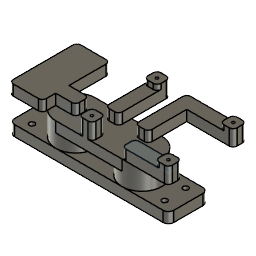
Halterung_Raspberry_Pi_5_XL4015 (Autodesk Fusion 360 design; units mm, degrees)
part number: 2026-02-12-18-16-56-274
Autodesk Fusion 360 part; units mm, degrees
note: some values were not read from the file. Set by a fixed rule: which sketch regions a step uses.
sketch "Skizze1" plane through (0, 0, 0) normal (0, 0, 1) x (1, 0, 0)
  line L0 (-35, 20) -> (85, 20)
  line L1 (85, 20) -> (85, -10)
  line L2 (85, -10) -> (-35, -10)
  line L3 (-35, -10) -> (-35, 20)
  dimension "d1" = 120
  dimension "d2" = 30
  constraint horizontal L0
  constraint vertical L1
  constraint horizontal L2
  constraint vertical L3
  measures "d1" distance of L0.start L0.end
  measures "d2" distance of L0.start L2.end
extrude "Extrusion1" add sketch "Skizze1" along normal blind 8
sketch "Skizze2" plane through (0, 0, 8) normal (0, 0, 1) x (-1, 0, 0)
  line L0 (35, 10) -> (-85, 10)
  line L1 (-85, 10) -> (-85, -20)
  line L2 (-85, -20) -> (35, -20)
  line L3 (35, -20) -> (35, 10)
  point P0 (25, -12.9992)
  point P1 (24.845, 3)
  point P2 (-75, -12.9991)
  point P3 (-75.16, 3.0001)
  dimension "d5" = 100
  dimension "d6" = 16
  dimension "d7" = 16
  dimension "d8" = 10
  dimension "d9" = 10
  dimension "d10" = 7
  measures "d5" distance of P0 P2
  measures "d6" distance of P2 P3
  measures "d7" distance of P0 P1
  measures "d8" distance of L3 P0
  measures "d9" distance of L1 P2
  measures "d10" distance of L0 P1
hole "Bohrung1" at (-25, 12.9992, 8) at (-24.845, -3, 8) at (75, 12.9991, 8) at (75.16, -3.0001, 8) direction (0, 0, -1) diameter 4 depth 45 tip angle 118
sketch "Skizze3" plane through (0, 0, 8) normal (0, 0, 1) x (-1, 0, 0)
  circle A0 centre (-75, -12.9991) radius 2
  circle A1 centre (25, -12.9992) radius 2
  circle A2 centre (24.845, 3) radius 2
  circle A3 centre (-75.16, 3.0001) radius 2
  line L0 (35, 10) -> (-85, 10)
  line L1 (-85, 10) -> (-85, -20)
  line L2 (-85, -20) -> (35, -20)
  line L3 (35, -20) -> (35, 10)
  circle A4 centre (0, -5) radius 15
  circle A5 centre (-50, -5) radius 15
  dimension "d14" = 30
  dimension "d15" = 30
  dimension "d16" = 35
  dimension "d17" = 35
  measures "d14" diameter of A4
  measures "d15" diameter of A5
  measures "d16" distance of L3 A4.centre
  measures "d17" distance of L1 A5.centre
extrude "Extrusion2" add sketch "Skizze3" along normal blind 10 contours A4 | A5
sketch "Skizze4" plane through (0, 0, 18) normal (0, 0, 1) x (-1, 0, 0)
  circle A0 centre (0, -5) radius 15
sketch "Skizze5" plane through (0, 0, 18) normal (0, 0, 1) x (-1, 0, 0)
  line L0 (15, -20) -> (-65, -20)
  line L1 (-65, -20) -> (-65, 10)
  line L2 (-65, 10) -> (15, 10)
  line L3 (15, 10) -> (15, -20)
  constraint horizontal L0
  constraint vertical L1
  constraint horizontal L2
  constraint vertical L3
extrude "Extrusion3" add sketch "Skizze5" along normal blind 8
fillet "Abrundung1" radius 15 1 edges at (-15, -10, 22)
fillet "Abrundung2" radius 15 1 edges at (-15, 20, 22)
fillet "Abrundung3" radius 15 1 edges at (65, 20, 22)
fillet "Abrundung4" radius 15 1 edges at (65, -10, 22)
sketch "Skizze6" plane through (0, 0, 26) normal (0, 0, 1) x (-1, 0, 0)
  arc A0 (-50, 10) -> (-50, -20) centre (-50, -5) ccw
  line L0 (-50, -20) -> (0, -20)
  arc A1 (0, -20) -> (0, 10) centre (0, -5) ccw
  line L1 (0, 10) -> (-50, 10)
  line L2 (-50, 10) -> (-85, 10)
  line L3 (-85, 10) -> (-85, 0)
  line L4 (-85, 0) -> (-50, 0)
  line L5 (-50, 0) -> (-50, 10)
  dimension "d32" = 10
  constraint horizontal L2
  constraint vertical L3
  constraint horizontal L4
  constraint vertical L5
  constraint coincident A0.start L1.end
  measures "d32" distance of A0.start L4.end
extrude "Extrusion4" add sketch "Skizze6" along normal blind 8 contours A0 L4 L5 | A0 L2 L3 L4
fillet "Abrundung5" radius 3 1 edges at (50, 0, 30)
fillet "Abrundung6" radius 3 1 edges at (50, -10, 30)
sketch "Skizze7" plane through (0, 0, 34) normal (0, 0, 1) x (-1, 0, 0)
  line L0 (-85, 10) -> (-85, 0)
  line L1 (-85, 0) -> (-53, 0)
  arc A0 (-53, 0) -> (-50, 3) centre (-53, 3) ccw
  line L2 (-50, 3) -> (-50, 7)
  arc A1 (-50, 7) -> (-53, 10) centre (-53, 7) ccw
  line L3 (-53, 10) -> (-85, 10)
sketch "Skizze8" plane through (0, 0, 34) normal (0, 0, 1) x (-1, 0, 0)
  line L0 (-85, 10) -> (-75, 10)
  line L1 (-75, 10) -> (-75, 0)
  line L2 (-75, 0) -> (-85, 0)
  line L3 (-85, 0) -> (-85, 10)
  constraint horizontal L0
  constraint vertical L1
  constraint horizontal L2
  constraint vertical L3
extrude "Extrusion5" add sketch "Skizze8" along normal blind 4
fillet "Abrundung9" radius 3 1 edges at (85, -10, 32)
fillet "Abrundung10" radius 3 1 edges at (85, 0, 32)
sketch "Skizze9" plane through (0, 0, 26) normal (0, 0, 1) x (-1, 0, 0)
  line L0 (-50, 7) -> (-50, 3)
  arc A0 (-53, 0) -> (-50, 3) centre (-53, 3) ccw
  line L1 (-53, 0) -> (-64.1421, 0)
  arc A1 (-64.1421, 0) -> (-50, -20) centre (-50, -5) ccw
  line L2 (-50, -20) -> (0, -20)
  arc A2 (0, -20) -> (0, 10) centre (0, -5) ccw
  line L3 (0, 10) -> (-50, 10)
  arc A3 (-50, 10) -> (-52.0792, 9.8552) centre (-50, -5) ccw
  arc A4 (-50, 7) -> (-52.0792, 9.8552) centre (-53, 7) ccw
  line L4 (-50, -9.8054) -> (-40, -9.8054)
  line L5 (-40, -9.8054) -> (-40, -48.8054)
  line L6 (-40, -48.8054) -> (-50, -48.8054)
  line L7 (-50, -48.8054) -> (-50, -9.8054)
  line L8 (-50, -38.8054) -> (-85, -38.8054)
  line L9 (-85, -38.8054) -> (-85, -48.8054)
  line L10 (-85, -48.8054) -> (-50, -48.8054)
  line L11 (-50, -48.8054) -> (-50, -38.8054)
  point P0 (-80, 5)
  point P1 (-80, -44)
  dimension "d47" = 49
  dimension "d48" = 39
  dimension "d49" = 10
  constraint horizontal L4
  constraint vertical L5
  constraint horizontal L6
  constraint vertical L7
  constraint horizontal L8
  constraint vertical L9
  constraint horizontal L10
  constraint vertical L11
  constraint coincident L7 L8.start
  measures "d47" distance of P0 P1
  measures "d48" distance of L4.end L5.end
  measures "d49" distance of L8.end L9.end
extrude "Extrusion6" add sketch "Skizze9" along normal blind 8 contours L2 L4 L5 L7 | L2 L5 L6 L7 L11 | L7 L8 L9 L10 L11
sketch "Skizze10" plane through (0, 0, 34) normal (0, 0, 1) x (-1, 0, 0)
  line L0 (-50, -38.8054) -> (-85, -38.8054)
  line L1 (-85, -38.8054) -> (-85, -48.8054)
  line L2 (-85, -48.8054) -> (-40, -48.8054)
  line L3 (-40, -48.8054) -> (-40, -9.8054)
  line L4 (-40, -9.8054) -> (-50, -9.8054)
  line L5 (-50, -9.8054) -> (-50, -38.8054)
  line L6 (-85, -38.8054) -> (-75.0603, -38.8054)
  line L7 (-75.0603, -38.8054) -> (-75.0603, -48.8054)
  line L8 (-75.0603, -48.8054) -> (-85, -48.8054)
  line L9 (-85, -48.8054) -> (-85, -38.8054)
  line L10 (-50, -38.8054) -> (-17, -38.8054)
  line L11 (-17, -38.8054) -> (-17, -49)
  line L12 (-17, -49) -> (-50, -49)
  line L13 (-50, -49) -> (-50, -38.8054)
  constraint horizontal L6
  constraint vertical L7
  constraint horizontal L8
  constraint vertical L9
  constraint coincident L2 L7.end
  constraint coincident L0.end L1.start
  constraint horizontal L10
  constraint vertical L11
  constraint horizontal L12
  constraint vertical L13
  constraint coincident L0.start L5.end
extrude "Extrusion7" add sketch "Skizze10" along normal blind 4 contours L0 L1 L2 L6 L7 L8 L9
fillet "Abrundung11" radius 3 1 edges at (85, 48.8054, 32)
fillet "Abrundung12" radius 3 1 edges at (85, 38.8054, 32)
fillet "Abrundung13" radius 3 1 edges at (40, 48.8054, 30)
fillet "Abrundung14" radius 3 1 edges at (40, 9.8054, 30)
fillet "Abrundung15" radius 3 1 edges at (50, 9.8054, 30)
sketch "Skizze11" plane through (0, 0, 26) normal (0, 0, 1) x (-1, 0, 0)
  line L0 (-40, -12.8054) -> (-40, -20)
  line L1 (-40, -20) -> (0, -20)
  arc A0 (0, -20) -> (0, 10) centre (0, -5) ccw
  line L2 (0, 10) -> (-50, 10)
  arc A1 (-50, 10) -> (-52.0792, 9.8552) centre (-50, -5) ccw
  arc A2 (-50, 7) -> (-52.0792, 9.8552) centre (-53, 7) ccw
  line L3 (-50, 7) -> (-50, 3)
  arc A3 (-53, 0) -> (-50, 3) centre (-53, 3) ccw
  line L4 (-53, 0) -> (-64.1421, 0)
  arc A4 (-64.1421, 0) -> (-50, -20) centre (-50, -5) ccw
  line L5 (-50, -20) -> (-50, -12.8054)
  arc A5 (-47, -9.8054) -> (-50, -12.8054) centre (-47, -12.8054) ccw
  line L6 (-47, -9.8054) -> (-43, -9.8054)
  arc A6 (-40, -12.8054) -> (-43, -9.8054) centre (-43, -12.8054) ccw
  line L7 (-27.3274, 10) -> (-17.3274, 10)
  line L8 (-17.3274, 10) -> (-17.3274, 0)
  line L9 (-17.3274, 0) -> (-27.3274, 0)
  line L10 (-27.3274, 0) -> (-27.3274, 10)
  point P0 (-80.3274, 5)
  point P1 (-22.3274, 5)
  dimension "d64" = 58
  dimension "d65" = 10
  dimension "d67" = 5
  constraint horizontal L7
  constraint vertical L8
  constraint horizontal L9
  constraint vertical L10
  constraint coincident L2 L7.start
  measures "d64" distance of P0 P1
  measures "d65" distance of L7.start L7.end
  measures "d67" distance of P1 L10
extrude "Extrusion8" add sketch "Skizze11" along normal blind 12 contours L2 L7 L8 L9 L10
fillet "Abrundung16" radius 3 1 edges at (17.3274, 0, 32)
fillet "Abrundung17" radius 3 1 edges at (27.3274, 0, 32)
fillet "Abrundung18" radius 3 1 edges at (27.3274, -10, 32)
fillet "Abrundung19" radius 3 1 edges at (17.3274, -10, 32)
sketch "Skizze13" plane through (0, 0, 26) normal (0, 0, 1) x (-1, 0, 0)
  line L0 (-17.3274, 7) -> (-17.3274, 3)
  arc A0 (-20.3274, 0) -> (-17.3274, 3) centre (-20.3274, 3) ccw
  line L1 (-20.3274, 0) -> (-24.3274, 0)
  arc A1 (-27.3274, 3) -> (-24.3274, 0) centre (-24.3274, 3) ccw
  line L2 (-27.3274, 3) -> (-27.3274, 7)
  arc A2 (-24.3274, 10) -> (-27.3274, 7) centre (-24.3274, 7) ccw
  line L3 (-24.3274, 10) -> (-50, 10)
  arc A3 (-50, 10) -> (-52.0792, 9.8552) centre (-50, -5) ccw
  arc A4 (-50, 7) -> (-52.0792, 9.8552) centre (-53, 7) ccw
  line L4 (-50, 7) -> (-50, 3)
  arc A5 (-53, 0) -> (-50, 3) centre (-53, 3) ccw
  line L5 (-53, 0) -> (-64.1421, 0)
  arc A6 (-64.1421, 0) -> (-50, -20) centre (-50, -5) ccw
  line L6 (-50, -20) -> (-50, -12.8054)
  arc A7 (-47, -9.8054) -> (-50, -12.8054) centre (-47, -12.8054) ccw
  line L7 (-47, -9.8054) -> (-43, -9.8054)
  arc A8 (-40, -12.8054) -> (-43, -9.8054) centre (-43, -12.8054) ccw
  line L8 (-40, -12.8054) -> (-40, -20)
  line L9 (-40, -20) -> (0, -20)
  arc A9 (0, -20) -> (0, 10) centre (0, -5) ccw
  line L10 (0, 10) -> (-20.3274, 10)
  arc A10 (-17.3274, 7) -> (-20.3274, 10) centre (-20.3274, 7) ccw
  line L11 (-27.3274, -10.0422) -> (-17.3274, -10.0422)
  line L12 (-17.3274, -10.0422) -> (-17.3274, -49.0422)
  line L13 (-17.3274, -49.0422) -> (-27.3274, -49.0422)
  line L14 (-27.3274, -49.0422) -> (-27.3274, -10.0422)
  point P0 (-43, -48.8054)
  dimension "d83" = 4
  dimension "d84" = 39
  dimension "d85" = 39
  constraint horizontal L11
  constraint vertical L12
  constraint horizontal L13
  constraint vertical L14
  measures "d83" distance of A7.start L7.end
  measures "d84" distance of L7.end P0
  measures "d85" distance of L11.end L12.end
extrude "Extrusion10" add sketch "Skizze13" along normal blind 8 contours L9 L12 L13 L14 | L9 L11 L12 L14
sketch "Skizze14" plane through (0, 0, 34) normal (0, 0, 1) x (-1, 0, 0)
  line L0 (-27.3274, -49.0422) -> (-17.3274, -49.0422)
  line L1 (-17.3274, -49.0422) -> (-17.3274, -10.0422)
  line L2 (-17.3274, -10.0422) -> (-27.3274, -10.0422)
  line L3 (-27.3274, -10.0422) -> (-27.3274, -49.0422)
  line L4 (-27.3274, -39.1735) -> (-17.3274, -39.1735)
  line L5 (-17.3274, -39.1735) -> (-17.3274, -49.1735)
  line L6 (-17.3274, -49.1735) -> (-27.3274, -49.1735)
  line L7 (-27.3274, -49.1735) -> (-27.3274, -39.1735)
  dimension "d88" = 10
  constraint horizontal L4
  constraint vertical L5
  constraint horizontal L6
  constraint vertical L7
  constraint coincident L3 L4.start
  measures "d88" distance of L4.start L6.end
extrude "Extrusion11" add sketch "Skizze14" along normal blind 4 contours L0 L1 L3 L4 L5 L7
fillet "Abrundung20" radius 3 1 edges at (27.3274, 49.0422, 32)
fillet "Abrundung21" radius 3 1 edges at (17.3274, 49.0422, 32)
fillet "Abrundung22" radius 3 1 edges at (27.3274, 10.0422, 30)
fillet "Abrundung23" radius 3 1 edges at (17.3274, 10.0422, 30)
sketch "Skizze15" plane through (0, 0, 26) normal (0, 0, 1) x (-1, 0, 0)
  line L0 (-17.3274, -13.0422) -> (-17.3274, -20)
  line L1 (-17.3274, -20) -> (0, -20)
  arc A0 (0, -20) -> (0, 10) centre (0, -5) ccw
  line L2 (0, 10) -> (-20.3274, 10)
  arc A1 (-17.3274, 7) -> (-20.3274, 10) centre (-20.3274, 7) ccw
  line L3 (-17.3274, 7) -> (-17.3274, 3)
  arc A2 (-20.3274, 0) -> (-17.3274, 3) centre (-20.3274, 3) ccw
  line L4 (-20.3274, 0) -> (-24.3274, 0)
  arc A3 (-27.3274, 3) -> (-24.3274, 0) centre (-24.3274, 3) ccw
  line L5 (-27.3274, 3) -> (-27.3274, 7)
  arc A4 (-24.3274, 10) -> (-27.3274, 7) centre (-24.3274, 7) ccw
  line L6 (-24.3274, 10) -> (-50, 10)
  arc A5 (-50, 10) -> (-52.0792, 9.8552) centre (-50, -5) ccw
  arc A6 (-50, 7) -> (-52.0792, 9.8552) centre (-53, 7) ccw
  line L7 (-50, 7) -> (-50, 3)
  arc A7 (-53, 0) -> (-50, 3) centre (-53, 3) ccw
  line L8 (-53, 0) -> (-64.1421, 0)
  arc A8 (-64.1421, 0) -> (-50, -20) centre (-50, -5) ccw
  line L9 (-50, -20) -> (-50, -12.8054)
  arc A9 (-47, -9.8054) -> (-50, -12.8054) centre (-47, -12.8054) ccw
  line L10 (-47, -9.8054) -> (-43, -9.8054)
  arc A10 (-40, -12.8054) -> (-43, -9.8054) centre (-43, -12.8054) ccw
  line L11 (-40, -12.8054) -> (-40, -20)
  line L12 (-40, -20) -> (-27.3274, -20)
  line L13 (-27.3274, -20) -> (-27.3274, -13.0422)
  arc A11 (-24.3274, -10.0422) -> (-27.3274, -13.0422) centre (-24.3274, -13.0422) ccw
  line L14 (-24.3274, -10.0422) -> (-20.3274, -10.0422)
  arc A12 (-17.3274, -13.0422) -> (-20.3274, -10.0422) centre (-20.3274, -13.0422) ccw
  line L15 (-5, 0) -> (35, 0)
  line L16 (35, 0) -> (35, -10)
  line L17 (35, -10) -> (-5, -10)
  line L18 (-5, -10) -> (-5, 0)
  constraint horizontal L15
  constraint vertical L16
  constraint horizontal L17
  constraint vertical L18
extrude "Extrusion12" add sketch "Skizze15" along normal blind 8 contours A0 L15 L17 L18 | A0 L15 L16 L17
sketch "Skizze16" plane through (0, 0, 0) normal (0, -1, 0) x (1, 0, 0)
  line L0 (-14.1421, 26) -> (5, 26)
  line L1 (5, 26) -> (5, 34)
  line L2 (5, 34) -> (-35, 34)
  line L3 (-35, 34) -> (-35, 26)
  line L4 (-35, 26) -> (-14.1421, 26)
  line L5 (-35, 34) -> (-10, 34)
  line L6 (-10, 34) -> (-10, 26)
  line L7 (-10, 26) -> (-35, 26)
  line L8 (-35, 26) -> (-35, 34)
  constraint horizontal L5
  constraint vertical L6
  constraint horizontal L7
  constraint vertical L8
  constraint coincident L0 L6.end
  constraint coincident L2.end L3.start
extrude "Extrusion13" add sketch "Skizze16" along normal blind 10 contours L0 L2 L3 L4 L5 L6 L7 L8
sketch "Skizze17" plane through (0, 10, 0) normal (0, 1, 0) x (-1, 0, 0)
  line L0 (14.1421, 26) -> (35, 26)
  line L1 (35, 26) -> (35, 34)
  line L2 (35, 34) -> (-5, 34)
  line L3 (-5, 34) -> (-5, 26)
  line L4 (-5, 26) -> (14.1421, 26)
  line L5 (35, 34) -> (10, 34)
  line L6 (10, 34) -> (10, 26)
  line L7 (10, 26) -> (35, 26)
  line L8 (35, 26) -> (35, 34)
  constraint horizontal L5
  constraint vertical L6
  constraint horizontal L7
  constraint vertical L8
  constraint coincident L1.end L2.start
extrude "Extrusion14" add sketch "Skizze17" along normal blind 31 contours L0 L1 L2 L4 L5 L6 L7 L8
fillet "Abrundung24" radius 3 1 edges at (-10, 41, 30)
fillet "Abrundung25" radius 3 1 edges at (-35, 41, 30)
fillet "Abrundung26" radius 3 1 edges at (-35, -10, 30)
fillet "Abrundung27" radius 3 1 edges at (-10, -10, 30)
fillet "Abrundung28" radius 3 1 edges at (5, 0, 30)
fillet "Abrundung29" radius 3 1 edges at (5, 10, 30)
fillet "Abrundung30" radius 3 1 edges at (75, -10, 36)
fillet "Abrundung31" radius 3 1 edges at (75, 0, 36)
fillet "Abrundung32" radius 3 1 edges at (75.0603, 48.8054, 36)
fillet "Abrundung33" radius 3 1 edges at (75.0603, 38.8054, 36)
fillet "Abrundung34" radius 4 4 edges at (85, -10, 4) (85, 20, 4) (-35, -10, 4) (-35, 20, 4)
fillet "Abrundung35" radius 3 2 edges at (27.3274, 39.1735, 36) (17.3274, 39.1735, 36)
sketch "Skizze18" plane through (0, 0, 38) normal (0, 0, 1) x (-1, 0, 0)
  arc A0 (-17.3274, -42.1735) -> (-20.3274, -39.1735) centre (-20.3274, -42.1735) ccw
  line L0 (-20.3274, -39.1735) -> (-24.3274, -39.1735)
  arc A1 (-24.3274, -39.1735) -> (-27.3274, -42.1735) centre (-24.3274, -42.1735) ccw
  line L1 (-27.3274, -42.1735) -> (-27.3274, -46.0422)
  arc A2 (-27.3274, -46.0422) -> (-24.3274, -49.0422) centre (-24.3274, -46.0422) ccw
  line L2 (-24.3274, -49.0422) -> (-20.3274, -49.0422)
  arc A3 (-20.3274, -49.0422) -> (-17.3274, -46.0422) centre (-20.3274, -46.0422) ccw
  line L3 (-17.3274, -46.0422) -> (-17.3274, -42.1735)
  line L4 (-27.3274, 7) -> (-27.3274, 3)
  line L5 (-24.3274, 0) -> (-20.3274, 0)
  line L6 (-75, 3) -> (-75, 7)
  line L7 (-85, 0) -> (-53, 0)
  line L8 (-78.0603, -38.8054) -> (-82, -38.8054)
  line L9 (-82, -48.8054) -> (-78.0603, -48.8054)
  line L10 (-75.0603, -45.8054) -> (-75.0603, -41.8054)
  point P0 (-22.3274, -44.0422)
  point P1 (-22.3274, 5)
  point P2 (-80, 5)
  point P3 (-80.0603, -43.8054)
  dimension "d129" = 5
  dimension "d130" = 5
  dimension "d131" = 5
  dimension "d132" = 5
  dimension "d133" = 5
  dimension "d134" = 5
  dimension "d135" = 5
  dimension "d136" = 5
  dimension "d137" = 5
  measures "d129" distance of L2 P0
  measures "d130" distance of L3 P0
  measures "d131" distance of P1 L4
  measures "d132" distance of P1 L5
  measures "d133" distance of P2 L6
  measures "d134" distance of P2 L7
  measures "d135" distance of P3 L8
  measures "d136" distance of P3 L9
  measures "d137" distance of P3 L10
hole "Bohrung2" at (22.3274, -5, 38) at (22.3274, 44.0422, 38) at (80.0603, 43.8054, 38) at (80, -5, 38) direction (0, 0, -1) diameter 2 depth 3 tip angle 180
